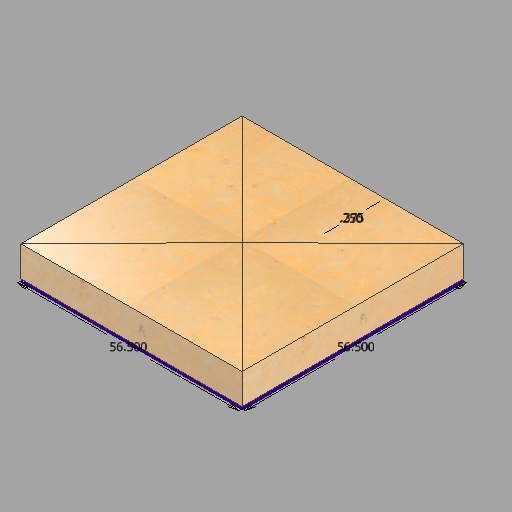
# Autodesk Inventor part: D - Cap - 2
Saved by Autodesk Inventor 2022.2 (Build 262287010, 287A)
## iProperties
RuleStatus: InUse
Created: 2022-03-23
Part Number: D - Cap - 2
Material: Granite, Cut, Polished
Document SubType Name: Modeling
Designer: awelt
Mass: 1.10578e+06 g
Surface Area: 53207.2 cm^2
Volume: 409547 cm^3
Density: 2.7 g/cm^3
Appearance: Amber Select
AfterDocSave0: Convert in3 volume to ft3
in3 to ft3: 14.46
TEST: 14.463
Author: awelt
Autodesk Inventor part; units mm, degrees
ref_plane "YZ Plane" through (0, 0, 0) normal (1, 0, 0) x (0, 1, 0)
ref_plane "XZ Plane" through (0, 0, 0) normal (0, 1, 0) x (-1, 0, 0)
ref_plane "XY Plane" through (0, 0, 0) normal (0, 0, 1) x (1, 0, 0)
sketch "Sketch1" plane through (0, 0, 0) normal (0, 1, 0) x (-1, 0, 0)
  line L0 (717.55, -717.55) -> (-717.55, -717.55)
  line L1 (-717.55, -717.55) -> (-717.55, 717.55)
  line L2 (-717.55, 717.55) -> (717.55, 717.55)
  line L3 (717.55, 717.55) -> (717.55, -717.55)
  line L4 (717.55, -717.55) -> (-717.55, 717.55) construction
  line L5 (-717.55, -717.55) -> (717.55, 717.55) construction
  line L6 (-708.025, -708.025) -> (708.025, -708.025)
  line L7 (708.025, -708.025) -> (708.025, 708.025)
  line L8 (708.025, 708.025) -> (-708.025, 708.025)
  line L9 (-708.025, 708.025) -> (-708.025, -708.025)
  line L10 (701.675, -701.675) -> (-701.675, -701.675)
  line L11 (-701.675, -701.675) -> (-701.675, 701.675)
  line L12 (-701.675, 701.675) -> (701.675, 701.675)
  line L13 (701.675, 701.675) -> (701.675, -701.675)
  point P0 (0, 0)
  dimension "d0" = 1435.1
  dimension "d1" = 1435.1
  dimension "d2" = 9.525
  dimension "d3" = 6.35
  constraints: 28 end point, 6 parallel, 3 perpendicular, 2 midpoint, 1 horizontal, 6 other
  measures "d0" distance of L1.end L2.end
  measures "d1" distance of L0.end L1.end
  measures "d2" distance between parallel lines of L0 L6
  measures "d3" distance between parallel lines of L6 L10
extrude "Extrusion1" add sketch "Sketch1" along normal blind 215.9 contours L0 L1 L2 L3 | L9 L8 L7 L6 | L10 L11 L12 L13
sketch "Sketch2" plane through (-717.55, 0, 717.55) normal (0, 0, 1) x (1, 0, 0)
  line L0 (0, 0) -> (1435.1, 0) projected
  line L1 (1435.1, 0) -> (1435.1, 215.9) projected
  line L2 (0, 215.9) -> (1435.1, 215.9) projected
  line L3 (0, 0) -> (0, 215.9) projected
  line L4 (0, 215.9) -> (1435.1, 215.9) projected
  line L5 (717.55, 215.9) -> (0, 209.55)
  line L6 (0, 215.9) -> (0, 209.55)
  line L7 (0, 0) -> (0, 215.9) projected
  line L8 (0, 215.9) -> (717.55, 215.9)
  line L9 (717.55, 215.9) -> (1435.1, 215.9)
  line L10 (1435.1, 0) -> (1435.1, 215.9) projected
  line L11 (1435.1, 215.9) -> (1435.1, 209.55)
  line L12 (1435.1, 209.55) -> (717.55, 215.9)
  point P0 (717.55, 0)
  dimension "d6" = 6.35
  dimension "d7" = 6.35
  constraints: 12 end point, 3 collinear, 2 point on line, 1 midpoint
  measures "d6" distance of L5.end L2.start
  measures "d7" distance of L11.end L1.end
sketch "Sketch3" plane through (717.55, 0, 717.55) normal (1, 0, 0) x (0, 0, -1)
  line L0 (0, 0) -> (1435.1, 0) projected
  line L1 (1435.1, 0) -> (1435.1, 215.9) projected
  line L2 (0, 215.9) -> (1435.1, 215.9) projected
  line L3 (0, 0) -> (0, 215.9) projected
  line L4 (0, 215.9) -> (1435.1, 215.9) projected
  line L5 (717.55, 215.9) -> (0, 209.55)
  line L6 (0, 0) -> (0, 215.9) projected
  line L7 (0, 215.9) -> (0, 209.55)
  line L8 (0, 215.9) -> (717.55, 215.9)
  line L9 (717.55, 215.9) -> (1435.1, 215.9)
  line L10 (1435.1, 0) -> (1435.1, 215.9) projected
  line L11 (1435.1, 215.9) -> (1435.1, 209.55)
  line L12 (1435.1, 209.55) -> (717.55, 215.9)
  point P0 (717.55, 0)
  point P1 (0, 209.55)
  dimension "d8" = 6.35
  dimension "d9" = 6.35
  constraints: 12 end point, 4 point on line, 2 collinear, 1 midpoint
  measures "d8" distance of L5.end L2.start
  measures "d9" distance of L11.end L1.end
extrude "Extrusion2" cut sketch "Sketch2" against normal through all contours L3 L2 L5 | L12 L2 L1
extrude "Extrusion3" cut sketch "Sketch3" against normal through all contours L3 L2 L5 | L12 L2 L1
extrude "Extrusion4" cut sketch "Sketch1" along normal blind 19.05 contours L9 L8 L7 L6
extrude "Extrusion5" cut sketch "Sketch1" along normal blind 12.7
body "Solid1"
